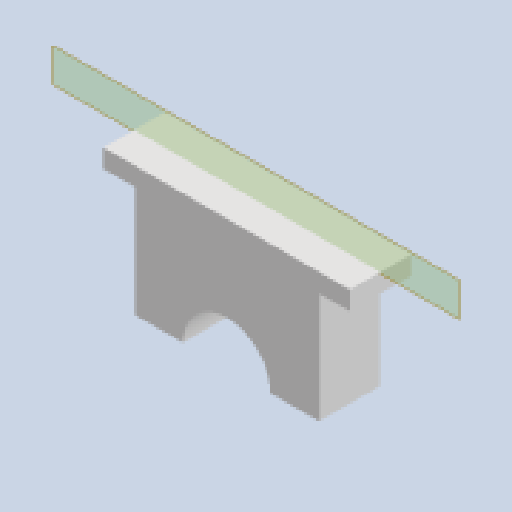
# Autodesk Inventor part: цили
Saved by Autodesk Inventor 2024.2 (Build 282272000, 272)
## iProperties
Created: 2025-11-23
Part Number: цили
Material: Типовые
Document SubType Name: Modeling
Designer: katya_notebook
Density: 1 g/cm^3
Appearance: По умолчанию
Author: katya_notebook
Autodesk Inventor part; units mm, degrees
ref_plane "YZ Plane" through (0, 0, 0) normal (1, 0, 0) x (0, 1, 0)
ref_plane "XZ Plane" through (0, 0, 0) normal (0, 1, 0) x (-1, 0, 0)
ref_plane "XY Plane" through (0, 0, 0) normal (0, 0, 1) x (1, 0, 0)
ref_plane "РабПлоскость2" through (-434.0611, 188.1702, -199.3103) normal (0, 0, -1) x (-1, 0, 0)
sketch "Эскиз2" plane through (-434.0611, 188.1702, -199.3103) normal (0, 0, -1) x (-1, 0, 0)
  circle A0 centre (-30.2445, -26) radius 2.5 projected
  circle A1 centre (-30.2445, -26) radius 2.5
  circle A2 centre (-30.2445, -26) radius 7.1
  line L0 (-60, -5) -> (0, -5) projected
  line L1 (-30.2445, -26) -> (-30.2445, -50.8115)
  line L2 (-30.2445, -50.8115) -> (-30.2445, 7.1034)
  line L3 (-30.2445, -5) -> (-50.2445, -5)
  line L4 (-50.2445, -5) -> (-50.2445, -8)
  line L5 (-50.2445, -8) -> (-45.2445, -8)
  circle A3 centre (-30.2445, -26) radius 15
  line L6 (-45.2445, -26) -> (-45.2445, -8)
  line L7 (-45.2445, -26) -> (-30.2445, -26)
  line L8 (-30.2445, -5) -> (-10.2445, -5)
  line L9 (-10.2445, -5) -> (-10.2445, -8)
  line L10 (-10.2445, -8) -> (-15.2445, -8)
  line L11 (-15.2445, -26) -> (-15.2445, -8)
  line L12 (-15.2445, -26) -> (-30.2445, -26)
  point P0 (-434.0611, -188.1702)
  point P1 (-37.3445, -26)
  point P2 (-23.1445, -26)
  point P3 (-10.2445, -5)
  dimension "d5" = 30
  dimension "d1" = 14.2
  dimension "d2" = 20
  dimension "d3" = 3
  constraints: 24 end point, 4 point on line, 4 symmetric about line, 3 coincident, 3 vertical, 2 centre point, 2 horizontal, 1 concentric, 1 horizontal alignment, 2 other
  measures "d1" diameter of A2
  measures "d2" distance of L3.start L3.end
  measures "d3" distance of L3.end L4.end
extrude "Выдавливание1" add sketch "Эскиз2" along normal mid plane 10 contours A2 L2 A3 L12 | A2 L7 A3 L2 | A3 L2 L0 L9 L10 L11 | A3 L6 L5 L4 L0 L2
